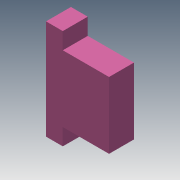
# Autodesk Inventor part: servodrzak1
Saved by Autodesk Inventor 2013 (Build 170138000, 138)
## iProperties
Created: 2013-01-30
Part Number: servodrzak1
Material: Generic
Document SubType Name: Modeling
Designer: idle-rug
Density: 1 g/cm^3
Author: idle-rug
Autodesk Inventor part; units mm, degrees
ref_plane "YZ Plane" through (0, 0, 0) normal (1, 0, 0) x (0, 1, 0)
ref_plane "XZ Plane" through (0, 0, 0) normal (0, 1, 0) x (-1, 0, 0)
ref_plane "XY Plane" through (0, 0, 0) normal (0, 0, 1) x (1, 0, 0)
sketch "Sketch2" plane through (0, 0, 0) normal (0, 1, 0) x (-1, 0, 0)
  line L0 (18.95, -27.5) -> (18.95, 27.5)
  line L1 (-18.95, -27.5) -> (18.95, 27.5) construction
  line L2 (18.95, -27.5) -> (-18.95, 27.5) construction
  line L3 (8.85, -27.5) -> (8.85, 27.5)
  line L4 (18.95, -30) -> (18.95, 30)
  line L5 (-18.95, -30) -> (18.95, 30) construction
  line L6 (18.95, -30) -> (-18.95, 30) construction
  line L7 (8.85, -30) -> (8.85, -20)
  line L8 (8.85, -20) -> (-18.95, -20)
  line L9 (8.85, 30) -> (8.85, 20)
  line L10 (8.85, 20) -> (-18.95, 20)
  line L11 (18.95, -30) -> (8.85, -30)
  line L12 (18.95, 30) -> (8.85, 30)
  line L13 (-18.95, -20) -> (-18.95, 20)
  point P0 (0, 0)
  dimension "d6" = 37.9
  dimension "d7" = 55
  dimension "d9" = 60
  dimension "d10" = 10
  dimension "d11" = 10
  constraints: 28 end point, 4 midpoint, 2 parallel, 2 point on line, 1 perpendicular
  measures "d6" distance of L2.end L0.end
  measures "d7" distance of L0.end L0.start
  measures "d9" distance of L4.end L4.start
  measures "d10" distance of L7.start L7.end
  measures "d11" distance of L9.start L9.end
extrude "Extrusion1" add sketch "Sketch2" along normal blind 15
body "Solid1"
